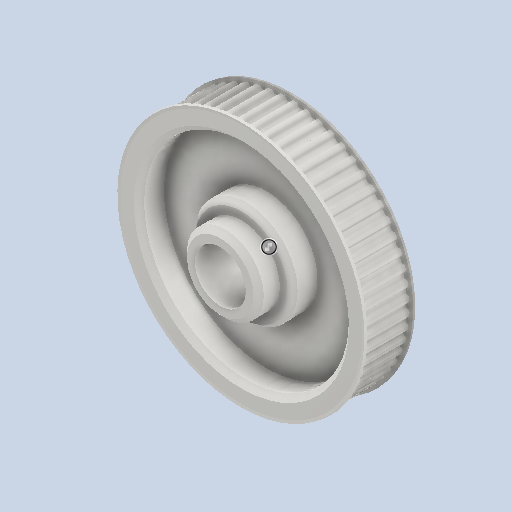
# Autodesk Inventor part: Synchroniczne koło pasowe1
Saved by Autodesk Inventor 2023 (Build 270158000, 158)
## iProperties
CustomPartVersion: 1
Created: 2023-04-25
Part Number: Synchroniczne koło pasowe1
Material: Steel
Document SubType Name: Modeling
Designer: krzys
Density: 7.85 g/cm^3
Appearance: Steel
Mass: 735.634 g
Surface Area: 278.842 cm^2
Volume: 93.7114 cm^3
Author: krzys
Autodesk Inventor part; units mm, degrees
ref_plane "YZ Plane" through (0, 0, 0) normal (1, 0, 0) x (0, 1, 0)
ref_plane "XZ Plane" through (0, 0, 0) normal (0, 1, 0) x (-1, 0, 0)
ref_plane "XY Plane" through (0, 0, 0) normal (0, 0, 1) x (1, 0, 0)
sketch "Szkic koła pasowego" plane through (0, 0, 0) normal (0, 0, 1) x (1, 0, 0)
  circle A0 centre (0, 0) radius 47.7465 construction
  circle A1 centre (0, 0) radius 47.2465
  circle A2 centre (0, 0) radius 45.9965
  line L0 (-1.4722, 47.2235) -> (-0.9, 45.9965)
  line L1 (-0.9, 45.9965) -> (0.9, 45.9965)
  line L2 (0.9, 45.9965) -> (1.4722, 47.2235)
  line L3 (0, 0) -> (0, 47.2465) construction
  circle A3 centre (0, 0) radius 10
  circle A4 centre (0, 0) radius 15
  circle A5 centre (0, 0) radius 20
  circle A6 centre (0, 0) radius 40
  point P0 (0, 45.9965)
  dimension "d0" = 95.493
  dimension "d1" = 0.5
  dimension "d2" = 1.25
  dimension "d3" = 50
  dimension "d4" = 1.8
  dimension "d17" = 20
  dimension "d18" = 30
  dimension "d26" = 40
  dimension "d27" = 80
  constraints: 8 end point, 7 coincident, 6 centre point, 3 point on circle, 1 horizontal, 1 midpoint, 1 point on line, 1 vertical, 1 vertical alignment, 3 other
  measures "d0" diameter of A0
  measures "d1" radial gap between concentric circles of A0 A1
  measures "d3" angle of L2 L0
  measures "d4" distance of L0.end L1.end
  measures "d17" diameter of A3
  measures "d18" diameter of A4
  measures "d26" diameter of A5
  measures "d27" diameter of A6
extrude "Bryła podstawowa" add sketch "Szkic koła pasowego" along normal mid plane 17.5 contours A2 | A1 L0 L1 L2 | L2 L1 L0 A1 | A3 | A4 | A5 | A6
extrude "Ząb" cut sketch "Szkic koła pasowego" along normal through all both and the other way through all contours L2 L1 L0 A1 picked at (0, 46.8281)
fillet "Fillet" radius 0.4 2 edges at (0.9, 45.9965, 0) (-0.9, 45.9965, 0)
fillet "Fillet" radius 0.6 4 edges at (-1.4722, 47.2235, 4.375) (-1.4722, 47.2235, -4.375) (1.4722, 47.2235, 4.375) (1.4722, 47.2235, -4.375)
pattern_circular "Zęby" count 60 over 360 about axis through (0, 0, -10) along (0, 0, 1) of "Ząb", "Fillet"
pulley flange "Obrzeże lewe" diameter 94.493 height 1.2 thickness 1 bend angle 10 centre (0, 0, -8.75) toward (0, 0, -1)
pulley flange "Obrzeże prawe" diameter 94.493 height 1.2 thickness 1 bend angle 10 centre (0, 0, 8.75) toward (0, 0, 1)
extrude "Wyciągnięcie proste3" cut sketch "Szkic koła pasowego" along normal through all both and the other way through all contours A3
extrude "Wyciągnięcie proste4" add sketch "Szkic koła pasowego" along normal blind 18 contours A4
chamfer "Faza1" distance 2 angle 45 1 edges at (-15, 0, 18)
extrude "Wyciągnięcie proste5" cut sketch "Szkic koła pasowego" along normal through all contours A6
chamfer "Faza2" distance 2 angle 45 2 edges at (-20, 0, 9.75) (-40, 0, 9.75)
equation "\"d1\" = da_a"
equation "\"d2\" = da_hg"
equation "\"d3\" = 2 * da_fi"
equation "\"d4\" = da_bw"
equation "\"d5\" = da_bf"
equation "\"d7\" = da_bf"
equation "\"d9\" = da_rb"
equation "\"d10\" = da_rt"
equation "\"da_pb\" = 5"
equation "\"da_fi\" = 25deg"
equation "\"da_hg\" = 1.25"
equation "\"da_bw\" = 1.8"
equation "\"da_rb\" = 0.4"
equation "\"da_rt\" = 0.6"
equation "\"da_a\" = 0.5"
equation "\"da_bf\" = 17.5"
equation "\"da_wf\" = 1"
equation "\"da_hf\" = 1.2"
body "Solid1"
